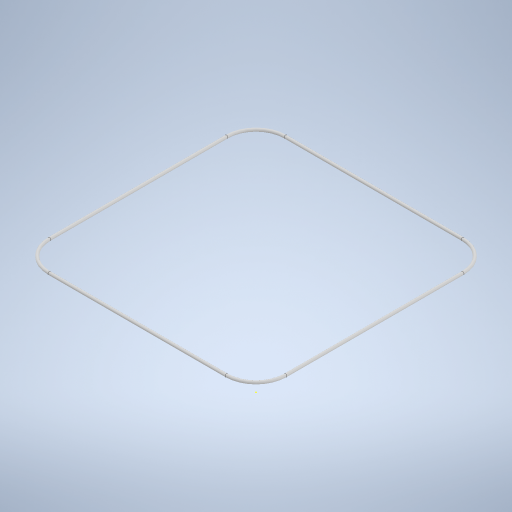
# Autodesk Inventor part: Riel
Saved by Autodesk Inventor 2024 (Build 280153000, 153)
## iProperties
Created: 2023-04-22
Part Number: Riel
Material: Genérico
Document SubType Name: Modeling
Designer: javie
Density: 1 g/cm^3
Appearance: Valor por defecto
Author: javie
Autodesk Inventor part; units mm, degrees
ref_plane "YZ Plane" through (0, 0, 0) normal (1, 0, 0) x (0, 1, 0)
ref_plane "XZ Plane" through (0, 0, 0) normal (0, 1, 0) x (-1, 0, 0)
ref_plane "XY Plane" through (0, 0, 0) normal (0, 0, 1) x (1, 0, 0)
sketch "Boceto1" plane through (0, 0, 0) normal (0, 1, 0) x (-1, 0, 0)
  point P0 (0, 0)
ref_plane "Plano de trabajo1" through (-3000, 0, 0) normal (-1, 0, 0) x (0, -1, 0)
sketch "Boceto2" plane through (-3000, 0, 0) normal (-1, 0, 0) x (0, -1, 0)
  circle A0 centre (0, 0) radius 25
  dimension "d11" = 50
  constraints: 1 centre point, 1 coincident
  measures "d11" diameter of A0
sketch3d "Boceto 3D1"
  line L0 (-3000, 0, 0) -> (-500, 0, 0)
  arc A0 (-500, 0, 0) -> (0, 0, -500) centre (-500, 0, -500) ccw
  line L1 (0, 0, -500) -> (0, 0, -3500)
  arc A1 (0, 0, -3500) -> (-500, 0, -4000) centre (-500, 0, -3500) ccw
  line L2 (-500, 0, -4000) -> (-3500, 0, -4000)
  arc A2 (-3500, 0, -4000) -> (-4000, 0, -3500) centre (-3500, 0, -3500) ccw
  line L3 (-4000, 0, -3500) -> (-4000, 0, -500)
  arc A3 (-4000, 0, -500) -> (-3500, 0, 0) centre (-3500, 0, -500) ccw
  line L4 (-3500, 0, 0) -> (-3000, 0, 0)
  dimension "d0" = 4000
  dimension "d1" = 4000
  dimension "d2" = 4000
  dimension "d5" = 500
  dimension "d6" = 500
  dimension "d7" = 3000
  dimension "d8" = 995
  dimension "d9" = 500
  dimension "d10" = 500
sweep "Barrido1" add profiles "Boceto2" path "Boceto 3D1"
equation "\"d5\" = d3"
equation "\"d6\" = d3"
equation "\"d10\" = d9"
equation "\"d3\" = 500"
